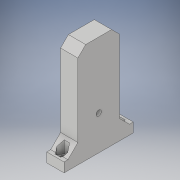
# Autodesk Inventor part: 000.209 - Крепеж крышки
Saved by Autodesk Inventor 2019 (Build 230136000, 136)
## iProperties
Created: 2020-04-11
Part Number: 000.209 - Крепеж крышки
Material: Типовые
Document SubType Name: Modeling
Designer: Петров Иван
Density: 1 g/cm^3
Appearance: По умолчанию
Author: Петров Иван
Autodesk Inventor part; units mm, degrees
ref_plane "YZ Plane" through (0, 0, 0) normal (1, 0, 0) x (0, 1, 0)
ref_plane "XZ Plane" through (0, 0, 0) normal (0, 1, 0) x (-1, 0, 0)
ref_plane "XY Plane" through (0, 0, 0) normal (0, 0, 1) x (1, 0, 0)
sketch "Эскиз1" plane through (0, 0, 0) normal (0, 1, 0) x (-1, 0, 0)
  line L0 (-5, 20) -> (5, 20)
  line L1 (5, 20) -> (5, -20)
  line L2 (5, -20) -> (-5, -20)
  line L3 (-5, -20) -> (-5, 20)
  line L4 (-5, 20) -> (5, -20) construction
  line L5 (5, 20) -> (-5, -20) construction
  point P0 (0, 0)
  dimension "d0" = 10
  dimension "d1" = 40
  constraints: 12 end point, 2 midpoint, 2 parallel, 1 horizontal, 1 perpendicular
  measures "d0" distance of L1.end L2.end
  measures "d1" distance of L0.end L1.end
extrude "Выдавливание1" add sketch "Эскиз1" along normal blind 3
sketch "Эскиз2" plane through (0, 3, 0) normal (0, 1, 0) x (1, 0, 0)
  line L0 (-5, 20) -> (-5, -20) projected
  line L1 (5, -12) -> (-5, -12)
  line L2 (-5, -12) -> (-5, 12)
  line L3 (-5, 12) -> (5, 12)
  line L4 (5, 12) -> (5, -12)
  line L5 (5, -12) -> (-5, 12) construction
  line L6 (-5, -12) -> (5, 12) construction
  point P0 (0, 0)
  dimension "d4" = 24
  constraints: 12 end point, 2 midpoint, 2 parallel, 1 horizontal, 1 perpendicular, 1 point on line
  measures "d4" distance of L1.end L2.end
extrude "Выдавливание2" add sketch "Эскиз2" along normal blind 55
sketch "Эскиз3" plane through (0, 3, 0) normal (0, 1, 0) x (1, 0, 0)
  circle A0 centre (0, -16) radius 1.5
  line L0 (-5, -12) -> (-5, -20) projected
  line L1 (-5, -20) -> (5, -20) projected
  point P0 (0, 0)
  dimension "d7" = 3
  dimension "d8" = 5
  dimension "d9" = 4
  constraints: 1 centre point
  measures "d7" diameter of A0
  measures "d8" distance from line of L0 A0.centre
  measures "d9" distance from line of L1 A0.centre
extrude "Выдавливание3" cut sketch "Эскиз3" against normal blind 20
mirror "Зеркальное отражение1" about plane through (0, 0, 0) normal (0, 0, 1) of "Выдавливание3"
sketch "Эскиз4" plane through (0, 3, 0) normal (0, 1, 0) x (1, 0, 0)
  circle A0 centre (0, -16) radius 1.5 projected
  line L0 (-3.1, -16) -> (-1.55, -13.3153)
  line L1 (-1.55, -13.3153) -> (1.55, -13.3153)
  line L2 (1.55, -13.3153) -> (3.1, -16)
  line L3 (3.1, -16) -> (1.55, -18.6847)
  line L4 (1.55, -18.6847) -> (-1.55, -18.6847)
  line L5 (-1.55, -18.6847) -> (-3.1, -16)
  line L6 (-5, -12) -> (5, -12) projected
  line L7 (5, -20) -> (-5, -20)
  line L8 (-5, -20) -> (-5, -12)
  line L9 (-5, -12) -> (5, -12)
  line L10 (5, -12) -> (5, -20)
  line L11 (5, -20) -> (-5, -12) construction
  line L12 (-5, -20) -> (5, -12) construction
  point P0 (0, 0)
  dimension "d12" = 6.2
  constraints: 24 end point, 2 midpoint, 2 parallel, 1 coincident, 1 horizontal, 1 perpendicular, 13 other
  measures "d12" distance of L2.end L0.start
extrude "Выдавливание4" add sketch "Эскиз4" along normal blind 2.5 contours L6 L10 L7 L8
mirror "Зеркальное отражение2" about plane through (0, 0, 0) normal (0, 0, 1) of "Выдавливание4"
sketch "Эскиз5" plane through (5, 0, 20) normal (1, 0, 0) x (0, 0, -1)
  circle A0 centre (20, 20) radius 1.5
  line L0 (40, 0) -> (0, 0) projected
  point P0 (20, 0)
  dimension "d16" = 3
  dimension "d29" = 20
  constraints: 1 centre point
  measures "d16" diameter of A0
  measures "d29" distance from line of A0.centre L0
extrude "Выдавливание5" cut sketch "Эскиз5" against normal blind 27.5
sketch "Эскиз6" plane through (-5, 0, -20) normal (-1, 0, 0) x (0, 0, 1)
  circle A0 centre (20, 20) radius 1.5 projected
  line L0 (20, 23.1) -> (22.6847, 21.55)
  line L1 (22.6847, 21.55) -> (22.6847, 18.45)
  line L2 (22.6847, 18.45) -> (20, 16.9)
  line L3 (20, 16.9) -> (17.3153, 18.45)
  line L4 (17.3153, 18.45) -> (17.3153, 21.55)
  line L5 (17.3153, 21.55) -> (20, 23.1)
  point P0 (20, 0)
  point P1 (0, 0)
  dimension "d20" = 6.2
  constraints: 12 end point, 2 coincident, 13 other
  measures "d20" distance of L2.end L0.start
extrude "Выдавливание6" cut sketch "Эскиз6" against normal blind 2.6
chamfer "Фаска1" distance 4.5 angle 45 2 edges at (0, 58, 12) (0, 58, -12)
chamfer "Фаска2" distance 5.75 angle 45 2 edges at (0, 5.5, 12) (0, 5.5, -12)
sketch "Эскиз7" plane through (0, 0, 0) normal (0, -1, 0) x (1, 0, 0)
  circle A0 centre (0, -16) radius 1.5 projected
  circle A1 centre (0, 16) radius 1.5 projected
  line L0 (5, 20) -> (-5, 20) projected
  line L1 (-5, 20) -> (-5, -20) projected
  line L2 (-5, -20) -> (5, -20) projected
  line L3 (5, -20) -> (5, 20) projected
  point P0 (0, 0)
